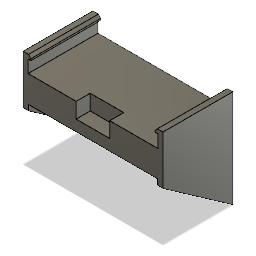
Sonar Bracket v2 (Autodesk Fusion 360 design; units mm, degrees)
Autodesk Fusion 360 part; units mm, degrees
sketch "Sketch1" plane through (0, 0, 0) normal (0, 1, 0) x (1, 0, 0)
  line L0 (25, -12.5) -> (-25, -12.5)
  line L1 (-25, -12.5) -> (-25, 12.5)
  line L2 (-25, 12.5) -> (25, 12.5)
  line L3 (25, 12.5) -> (25, -12.5)
  line L4 (25, -12.5) -> (-25, 12.5) construction
  line L5 (-25, -12.5) -> (25, 12.5) construction
  dimension "d1" = 25
  dimension "d2" = 50
  constraint perpendicular L0 L1
  constraint parallel L0 L2
  constraint parallel L1 L3
  constraint horizontal L0
  constraint coincident L4 origin
  constraint coincident L5 origin
  measures "d1" distance of L0.end L1.end
  measures "d2" distance of L1.end L2.end
extrude "Extrude1" add sketch "Sketch1" along normal blind 35
sketch "Sketch2" plane through (0, 0, 12.5) normal (0, 0, 1) x (1, 0, 0)
  line L0 (-25, 0) -> (25, 0)
  line L1 (25, 0) -> (25, 35)
  line L2 (25, 35) -> (-25, 35)
  line L3 (-25, 35) -> (-25, 0)
  line L4 (0, 0) -> (0, 11) construction
  line L5 (23, 35) -> (22.15, 34.1)
  line L6 (22.15, 34.1) -> (22.15, 33.5)
  line L7 (22.15, 33.5) -> (23.15, 33.5)
  line L8 (23.15, 33.5) -> (23.15, 29)
  line L9 (23.15, 29) -> (0, 29)
  line L10 (23, 35) -> (0, 35)
  line L11 (-25, 35) -> (25, 35)
  line L12 (-23.15, 33.5) -> (-23.15, 29)
  line L13 (-25, 0) -> (-25, 35)
  line L14 (-23, 35) -> (0, 35)
  line L15 (-22.15, 33.5) -> (-23.15, 33.5)
  line L16 (-22.15, 34.1) -> (-22.15, 33.5)
  line L17 (-23.15, 29) -> (0, 29)
  line L18 (-23, 35) -> (-22.15, 34.1)
  dimension "d5" = 46.3
  dimension "d6" = 1
  dimension "d7" = 1.5
  dimension "d8" = 0.6
  dimension "d9" = 2
  dimension "d10" = 4.5
  constraint coincident L4.start origin
  constraint perpendicular L0 L4
  constraint coincident L2 L5.start
  constraint perpendicular L2 L6
  constraint perpendicular L6 L7
  constraint perpendicular L7 L8
  constraint perpendicular L6 L9
  constraint midpoint L2 L10.end
  constraint symmetric L0.end L4 L0.start
  constraint symmetric L1.end L4 L2.end
  constraint symmetric L2.end L4 L1.end
  constraint symmetric L4 L5.start L14.start
  constraint symmetric L4 L5.end L16.start
  constraint symmetric L4 L6.end L15.start
  constraint symmetric L4 L7.end L12.start
  constraint symmetric L4 L8.end L12.end
  constraint symmetric L4 L9.end L17.end
  constraint symmetric L4 L10.end L14.end
  measures "d5" distance of L8 L12
  measures "d6" distance of L6.end L7.end
  measures "d7" distance of L7.end L10
  measures "d8" distance of L5.end L6.end
  measures "d9" distance of L5.start L1.end
  measures "d10" distance of L7.end L8.end
extrude "Extrude2" cut sketch "Sketch2" against normal through all contours L2 L5 L6 L7 L8 L9 L10 L11 L12 L14 L15 L16 L17 L18
sketch "Sketch3" plane through (0, 0, 12.5) normal (0, 0, 1) x (1, 0, 0)
  line L0 (23, 35) -> (22.15, 34.1)
  line L1 (22.15, 34.1) -> (22.15, 33.5)
  line L2 (22.15, 33.5) -> (23.15, 33.5)
  line L3 (23.15, 33.5) -> (23.15, 29)
  line L4 (23.15, 29) -> (-23.15, 29)
  line L5 (-23.15, 29) -> (-23.15, 33.5)
  line L6 (-23.15, 33.5) -> (-22.15, 33.5)
  line L7 (-22.15, 33.5) -> (-22.15, 34.1)
  line L8 (-22.15, 34.1) -> (-23, 35)
  line L9 (-23, 35) -> (-25, 35)
  line L10 (-25, 35) -> (-25, 0)
  line L11 (-25, 0) -> (25, 0)
  line L12 (25, 0) -> (25, 35)
  line L13 (25, 35) -> (23, 35)
  line L14 (6, 23.5) -> (-6, 23.5)
  line L15 (-6, 23.5) -> (-6, 34.5)
  line L16 (-6, 34.5) -> (6, 34.5)
  line L17 (6, 34.5) -> (6, 23.5)
  line L18 (6, 23.5) -> (-6, 34.5) construction
  line L19 (-6, 23.5) -> (6, 34.5) construction
  point P0 (0, 29)
  dimension "d12" = 12
  dimension "d13" = 11
  constraint perpendicular L14 L15
  constraint parallel L14 L16
  constraint parallel L15 L17
  constraint horizontal L14
  constraint coincident L18 P0
  constraint coincident L19 P0
  constraint midpoint L4 P0
  measures "d12" distance of L14.start L14.end
  measures "d13" distance of L14.start L16.end
extrude "Extrude3" cut sketch "Sketch3" against normal blind 5 contours L4 L14 L15 L17
sketch "Sketch4" plane through (25, 0, 0) normal (1, 0, 0) x (0, 0, -1)
  line L0 (-12.5, 0) -> (12.5, 0)
  line L1 (12.5, 0) -> (12.5, 35)
  line L2 (12.5, 35) -> (-12.5, 35)
  line L3 (-12.5, 35) -> (-12.5, 0)
  line L4 (-12.5, 17.5) -> (12.5, 0)
  line L5 (12.5, 0) -> (-12.5, 0)
  line L6 (-12.5, 0) -> (-12.5, 17.5)
  constraint midpoint L3 L4.start
  constraint coincident L0.end L1.start
  constraint coincident L0.start L3.end
extrude "Extrude4" cut sketch "Sketch4" against normal through all contours L0 L3 L4 L5 L6
sketch "Sketch5" plane through (0, 0, 12.5) normal (0, 0, 1) x (1, 0, 0)
  line L0 (-25, 17.5) -> (25, 17.5)
  line L1 (25, 17.5) -> (25, 35)
  line L2 (25, 35) -> (23, 35)
  line L3 (23, 35) -> (22.15, 34.1)
  line L4 (22.15, 34.1) -> (22.15, 33.5)
  line L5 (22.15, 33.5) -> (23.15, 33.5)
  line L6 (23.15, 33.5) -> (23.15, 29)
  line L7 (23.15, 29) -> (6, 29)
  line L8 (6, 29) -> (6, 23.5)
  line L9 (6, 23.5) -> (-6, 23.5)
  line L10 (-6, 23.5) -> (-6, 29)
  line L11 (-6, 29) -> (-23.15, 29)
  line L12 (-23.15, 29) -> (-23.15, 33.5)
  line L13 (-23.15, 33.5) -> (-22.15, 33.5)
  line L14 (-22.15, 33.5) -> (-22.15, 34.1)
  line L15 (-22.15, 34.1) -> (-23, 35)
  line L16 (-23, 35) -> (-25, 35)
  line L17 (-25, 35) -> (-25, 17.5)
  line L18 (23, 19.5) -> (-23, 19.5)
  line L19 (-23, 19.5) -> (-23, 0)
  line L20 (-23, 0) -> (23, 0)
  line L21 (23, 0) -> (23, 19.5)
  line L22 (23, 19.5) -> (-23, 0) construction
  line L23 (-23, 19.5) -> (23, 0) construction
  line L24 (-25, 0) -> (25, 0)
  line L25 (25, 17.5) -> (25, 0)
  line L26 (-25, 0) -> (-25, 17.5)
  point P0 (0, 9.75)
  dimension "d17" = 2
  dimension "d18" = 2
  dimension "d19" = 2
  constraint perpendicular L18 L19
  constraint parallel L18 L20
  constraint parallel L19 L21
  constraint horizontal L18
  constraint coincident L22 P0
  constraint coincident L23 P0
  constraint collinear L20 L24
  measures "d17" distance of L0 L18
  measures "d18" distance of L21 L25
  measures "d19" distance of L19 L26
extrude "Extrude5" cut sketch "Sketch5" against normal blind 21 contours L0 L18 L19 L21 | L0 L19 L20 L21 L24
sketch "Sketch6" plane through (0, 0, -8.5) normal (0, 0, 1) x (1, 0, 0)
  line L0 (-23, 2.8) -> (23, 2.8)
  line L1 (23, 2.8) -> (23, 19.5)
  line L2 (23, 19.5) -> (-23, 19.5)
  line L3 (-23, 19.5) -> (-23, 2.8)
  circle A0 centre (0, 9.5) radius 3.25
  line L4 (0, 0) -> (0, 14) construction
  dimension "d22" = 6.5
  dimension "d23" = 9.5
  constraint coincident L4.start origin
  constraint vertical L4
  constraint coincident A0.centre L4
  measures "d22" diameter of A0
  measures "d23" distance of L4.start A0.centre
extrude "Extrude6" cut sketch "Sketch6" against normal through all contours A0
